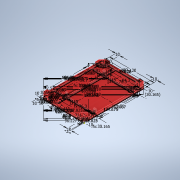
# Autodesk Inventor part: Prod5.2.1 - SKR1.4 Turbo Case Base
Saved by Autodesk Inventor 2021 (Build 250183000, 183)
## iProperties
Created: 2021-03-25
Part Number: Prod5.2.1 - SKR1.4 Turbo Case Base
Material: Generic
Document SubType Name: Modeling
Designer: alexr
Density: 1 g/cm^3
Appearance: Red
Author: alexr
Autodesk Inventor part; units mm, degrees
ref_plane "YZ Plane" through (0, 0, 0) normal (1, 0, 0) x (0, 1, 0)
ref_plane "XZ Plane" through (0, 0, 0) normal (0, 1, 0) x (-1, 0, 0)
ref_plane "XY Plane" through (0, 0, 0) normal (0, 0, 1) x (1, 0, 0)
sketch "Base Sketch" plane through (0, 0, 0) normal (0, 1, 0) x (-1, 0, 0)
  line L0 (10, 0) -> (110, 0)
  line L1 (120, -10) -> (120, -160)
  line L2 (110, -170) -> (10, -170)
  line L3 (0, -160) -> (0, -10)
  line L4 (86.3, -30.165) -> (2, -30.165) construction
  line L5 (2, -30.165) -> (2, -139.835) construction
  line L6 (2, -139.835) -> (86.3, -139.835) construction
  line L7 (86.3, -139.835) -> (86.3, -30.165) construction
  line L8 (82.3, -34.075) -> (6, -34.075) construction
  line L9 (6, -34.075) -> (6, -135.925) construction
  line L10 (6, -135.925) -> (82.3, -135.925) construction
  line L11 (82.3, -135.925) -> (82.3, -34.075) construction
  line L12 (0, -10) -> (10, 0)
  line L13 (120, -10) -> (110, 0)
  line L14 (120, -160) -> (110, -170)
  line L15 (0, -160) -> (10, -170)
  line L16 (100, 0) -> (100, -10)
  line L17 (120, -20) -> (110, -20)
  line L18 (100, -10) -> (110, -20)
  line L19 (120, -85) -> (0, -85) construction
  line L20 (60, 0) -> (60, -170) construction
  line L21 (100, -170) -> (100, -160)
  line L22 (120, -150) -> (110, -150)
  line L23 (100, -160) -> (110, -150)
  line L24 (20, 0) -> (20, -10)
  line L25 (0, -20) -> (10, -20)
  line L26 (20, -10) -> (10, -20)
  line L27 (20, -170) -> (20, -160)
  line L28 (20, -160) -> (10, -150)
  line L29 (0, -150) -> (10, -150)
  circle A0 centre (82.3, -34.075) radius 3
  circle A1 centre (6, -34.075) radius 3
  circle A2 centre (82.3, -135.925) radius 3
  circle A3 centre (6, -135.925) radius 3
  line L30 (82.8, -5) -> (82.8, -31.117)
  line L31 (80.3, -5) -> (80.3, -31.8389)
  line L32 (80.3, -36.3111) -> (80.3, -133.6889)
  line L33 (80.3, -138.1611) -> (80.3, -165)
  line L34 (82.8, -37.033) -> (82.8, -132.967)
  line L35 (82.8, -138.883) -> (82.8, -165)
  line L36 (79.5728, -35.325) -> (8.7272, -35.325)
  line L37 (79.5728, -32.825) -> (8.7272, -32.825)
  line L38 (85.0272, -35.325) -> (115, -35.325)
  line L39 (85.0272, -32.825) -> (115, -32.825)
  line L40 (8.7272, -134.675) -> (79.5728, -134.675)
  line L41 (85.0272, -134.675) -> (115, -134.675)
  line L42 (8.7272, -137.175) -> (79.5728, -137.175)
  line L43 (85.0272, -137.175) -> (115, -137.175)
  line L44 (80.3, -165) -> (12.0711, -165)
  line L45 (12.0711, -165) -> (5, -157.9289)
  line L46 (5, -157.9289) -> (5, -12.0711)
  line L47 (5, -12.0711) -> (12.0711, -5)
  line L48 (12.0711, -5) -> (80.3, -5)
  line L49 (82.8, -165) -> (107.9289, -165)
  line L50 (107.9289, -165) -> (115, -157.9289)
  line L51 (115, -157.9289) -> (115, -137.175)
  line L52 (82.8, -5) -> (107.9289, -5)
  line L53 (107.9289, -5) -> (115, -12.0711)
  line L54 (115, -12.0711) -> (115, -32.825)
  line L55 (115, -134.675) -> (115, -35.325)
  point P0 (0, 0)
  point P1 (120, -170)
  point P2 (120, 0)
  point P3 (0, -170)
  point P4 (110, -10)
  point P5 (110, -160)
  point P6 (10, -10)
  point P7 (10, -160)
  point P8 (20, -165)
  point P9 (100, -165)
  point P10 (115, -150)
  point P11 (115, -20)
  point P12 (100, -5)
  point P13 (20, -5)
  point P14 (5, -150)
  point P15 (5, -138.7534)
  point P16 (5, -133.0966)
  point P17 (5, -36.9034)
  point P18 (5, -31.2466)
  point P19 (5, -20)
  dimension "d109" = 6
  dimension "d0" = 120
  dimension "d1" = 170
  dimension "d12" = 84.3
  dimension "d13" = 109.67
  dimension "d14" = 76.3
  dimension "d15" = 101.85
  dimension "d16" = 3.91
  dimension "d17" = 3.91
  dimension "d18" = 4
  dimension "d19" = 4
  dimension "d20" = 2
  dimension "d21" = 30.165
  dimension "d22" = 30.165
  dimension "d82" = 10
  dimension "d83" = 10
  dimension "d84" = 10
  dimension "d85" = 10
  dimension "d88" = 10
  dimension "d90" = 10
  dimension "d91" = 10
  dimension "d93" = 10
  dimension "d94" = 190.9188
  dimension "d95" = 10
  dimension "d96" = 0
  dimension "d101" = 10
  dimension "d102" = 10
  dimension "d103" = 10
  dimension "d104" = 10
  dimension "d113" = 76.3
  dimension "d116" = 101.85
  dimension "d143" = 10
  dimension "d144" = 10
  dimension "d166" = 90
  dimension "d167" = 90
  dimension "d168" = 90
  dimension "d169" = 90
  dimension "d170" = 90
  dimension "d171" = 135
  dimension "d172" = 135
  dimension "d173" = 45
  dimension "d174" = 45
  dimension "d175" = 45
  dimension "d176" = 45
  dimension "d177" = 5
  dimension "d178" = 37.2
  dimension "d179" = 39.7
  dimension "d180" = 115
  dimension "d181" = 5
  dimension "d182" = 185.9188
  dimension "d183" = 9.1421
  dimension "d184" = 180.9188
  dimension "d185" = 2.5
  dimension "d186" = 104.35
  dimension "d187" = 101.85
  dimension "d188" = 27.825
  dimension "d189" = 132.175
  dimension "d190" = 12.825
  dimension "d191" = 160
  dimension "d192" = 115
  dimension "d193" = 115
  dimension "d194" = 82.8
  dimension "d195" = 82.8
  dimension "d196" = 80.3
  dimension "d197" = 80.3
  constraints: 112 end point, 24 parallel, 18 symmetric about line, 11 point on line, 5 horizontal, 4 midpoint, 4 perpendicular, 4 point on circle, 2 centre point, 2 vertical, 1 coincident, 1 line through centre, 24 other
  measures "d0" distance of point (120, -170) point (0, -170)
  measures "d1" distance of point (120, 0) point (120, -170)
  measures "d12" distance of L6.end L5.end
  measures "d13" distance of L5.end L4.end
  measures "d14" distance of L10.end L9.end
  measures "d15" distance of L9.end L8.end
  measures "d16" distance between parallel lines of L6 L10
  measures "d17" distance between parallel lines of L4 L8
  measures "d18" distance between parallel lines of L7 L11
  measures "d19" distance between parallel lines of L9 L5
  measures "d20" distance between parallel lines of L3 L5
  measures "d21" distance between parallel lines of L0 L4
  measures "d22" distance between parallel lines of L2 L6
  measures "d82" horizontal distance of L3.start L2.end
  measures "d83" horizontal distance of L3.end L0.start
  measures "d84" horizontal distance of L3.end L0.start
  measures "d85" horizontal distance of L3.start L2.end
  measures "d88" horizontal distance of L1.end L14.end
  measures "d90" distance from line of L0.end L1
  measures "d91" distance from line of L2.start L1
  measures "d93" distance from line of L13.end L1
  measures "d94" distance between parallel lines of L13 L15
  measures "d95" distance from line of point (110, 0) L1
  measures "d96" distance from line of point (110, 0) L13
  measures "d101" distance of L16.start L16.end
  measures "d102" distance of L17.start L17.end
  measures "d103" distance from line of L0.end L16
  measures "d104" distance from line of L1.start L17
  measures "d113" distance of point (82.3, -34.075) A1.centre
  measures "d116" distance of point (82.3, -34.075) point (82.3, -135.925)
  measures "d143" distance of point (110, -10) L1.start
  measures "d144" distance from line of L0 point (110, -10)
  measures "d166" angle of L48 L1
  measures "d167" angle of L37 L1
  measures "d168" angle of L36 L1
  measures "d169" angle of L40 L1
  measures "d170" angle of L42 L1
  measures "d171" angle of L54 L13
  measures "d172" angle of L55 L13
  measures "d173" angle of L30 L13
  measures "d174" angle of L34 L13
  measures "d175" angle of L31 L13
  measures "d176" angle of L32 L13
  measures "d177" distance between parallel lines of L51 L1
  measures "d178" distance between parallel lines of L35 L1
  measures "d179" distance between parallel lines of L33 L1
  measures "d180" distance between parallel lines of L46 L1
  measures "d181" distance between parallel lines of L50 L14
  measures "d182" distance between parallel lines of L47 L14
  measures "d183" distance between parallel lines of L18 L53
  measures "d184" distance between parallel lines of L53 L45
  measures "d185" distance between parallel lines of L39 L38
  measures "d186" distance between parallel lines of L39 L43
  measures "d187" distance between parallel lines of L39 L41
  measures "d188" distance between parallel lines of L39 L52
  measures "d189" distance between parallel lines of L39 L49
  measures "d190" distance between parallel lines of L25 L39
  measures "d191" distance between parallel lines of L48 L44
  measures "d192" distance from line of point (0, 0) L54
  measures "d193" distance from line of point (0, 0) L55
  measures "d194" distance from line of point (0, 0) L30
  measures "d195" distance from line of point (0, 0) L34
  measures "d196" distance from line of point (0, 0) L31
  measures "d197" distance from line of point (0, 0) L32
extrude "Main Body" add sketch "Base Sketch" against normal blind 1.5
extrude "Structure" add sketch "Base Sketch" along normal blind 3.5 contours L0 L16 L52 L30 A0 L31 L48 L24 | L25 L46 A1 A3 L29 L3 | L1 L22 L51 L43 A2 L41 L55 L38 A0 L39 L54 L17 | A0 L36 A1 L37 | L27 L44 L33 A2 L35 L49 L21 L2 | A3 L40 A2 L42 | A0 L34 A2 L32
extrude "Corners" add sketch "Base Sketch" along normal blind 8.5 contours L0 L24 L48 L47 L46 L25 L3 L12 | L0 L13 L1 L17 L54 L53 L52 L16 | L24 L26 L25 L46 L47 L48 | L52 L53 L54 L17 L18 L16 | L29 L46 L45 L44 L27 L2 L15 L3 | L29 L28 L27 L44 L45 L46 | L1 L14 L2 L21 L49 L50 L51 L22 | L51 L50 L49 L21 L23 L22
extrude "Board Standoffs" add sketch "Base Sketch" along normal blind 13 contours A0 | L46 A1 | A1 L46 | L46 A3 | A3 L46 | A2
hole "Standoff Hole" at (-6, 0, -34.075) at (-6, 0, -135.925) at (-82.3, 0, -135.925) at (-82.3, 0, -34.075) direction (0, -1, 0) diameter 2.5 end through all both
hole "Corner Hole" at (-110, 0, -10) at (-110, 0, -160) at (-10, 0, -10) at (-10, 0, -160) direction (0, -1, 0) diameter 4.5 end through all both
equation "\"d16\" = d17"
equation "\"d18\" = d19"
equation "\"d21\" = d22"
equation "\"d113\" = d14"
equation "\"d116\" = d15"
body "Solid2"
